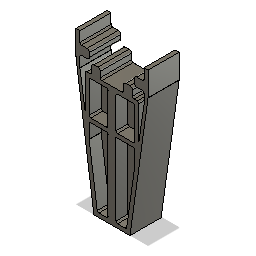
Tornado_Foot_75mm (Autodesk Fusion 360 design; units mm, degrees)
Autodesk Fusion 360 part; units mm, degrees
sketch "Sketch1" plane through (0, 0, 0) normal (0, 0, 1) x (1, 0, 0)
  line L0 (0, 0) -> (22.5, 0)
  line L1 (22.5, 0) -> (22.5, 95)
  line L2 (22.5, 95) -> (0, 95)
  line L3 (0, 95) -> (0, 0)
  line L4 (0, 95) -> (20, 95)
  line L5 (20, 95) -> (20, 75)
  line L6 (20, 75) -> (0, 75)
  line L7 (0, 75) -> (0, 95)
  line L8 (20, 95) -> (20, 85) construction
  line L9 (14, 87.75) -> (26, 87.75)
  line L10 (26, 87.75) -> (26, 82.25)
  line L11 (26, 82.25) -> (14, 82.25)
  line L12 (14, 82.25) -> (14, 87.75)
  line L13 (14, 87.75) -> (26, 82.25) construction
  line L14 (26, 87.75) -> (14, 82.25) construction
  line L15 (12.75, 81) -> (7.25, 81)
  line L16 (7.25, 81) -> (7.25, 69)
  line L17 (7.25, 69) -> (12.75, 69)
  line L18 (12.75, 69) -> (12.75, 81)
  line L19 (12.75, 81) -> (7.25, 69) construction
  line L20 (7.25, 81) -> (12.75, 69) construction
  line L21 (22.5, 80) -> (11.25, 0)
  line L22 (11.25, 0) -> (8.7744, 0.3481)
  line L23 (8.7744, 0.3481) -> (20, 75)
  line L24 (12.75, 75) -> (16.75, 75)
  line L25 (16.75, 75) -> (16.75, 53.3871)
  point P0 (20, 85)
  point P1 (10, 75)
  dimension "d1" = 5.5
  dimension "d2" = 12
  dimension "d3" = 12
  dimension "d4" = 5.5
  dimension "d5" = 22.5
  dimension "d6" = 95
  dimension "d7" = 20
  dimension "d8" = 20
  dimension "d28" = 2.5
  dimension "d29" = 4
  constraint horizontal L0
  constraint vertical L1
  constraint horizontal L2
  constraint vertical L3
  constraint coincident L0.start L3.end
  constraint horizontal L4
  constraint vertical L5
  constraint horizontal L6
  constraint vertical L7
  constraint midpoint L5 P0
  constraint perpendicular L9 L10
  constraint parallel L9 L11
  constraint parallel L10 L12
  constraint horizontal L9
  constraint coincident L13 P0
  constraint coincident L14 P0
  constraint coincident P0 L8.end
  constraint perpendicular L15 L16
  constraint parallel L15 L17
  constraint parallel L16 L18
  constraint horizontal L15
  constraint coincident L19 P1
  constraint coincident L20 P1
  constraint midpoint L6 P1
  constraint coincident L1 L21.start
  constraint midpoint L0 L21.end
  constraint perpendicular L21 L22
  constraint midpoint L18 L24.start
  constraint perpendicular L5 L24
  constraint vertical L25
  constraint coincident L23 L25.end
  measures "d1" distance of L9.end L10.end
  measures "d2" distance of L10.end L11.end
  measures "d3" distance of L15.end L16.end
  measures "d4" distance of L16.end L17.end
  measures "d5" distance of L0.start L0.end
  measures "d6" distance of L0.end L1.end
  measures "d7" distance of L4.end L5.end
  measures "d8" distance of L5.end L6.end
  measures "d28" distance of L21.end L22.end
  measures "d29" distance of L24.start L24.end
extrude "Extrude1" add sketch "Sketch1" along normal blind 10 contours L0 L3 L6 L16 L17 L18 L22 L23 L24 L25 | L1 L5 L11 L21 L22 L23 | L6 L15 L16 L18 | L6 L16 L17 L18 | L1 L5 L9 L11 | L1 L2 L5 L9 | L5 L9 L11 L12 makes body 1
fillet "Fillet1" [suppressed]
chamfer "Chamfer1" [suppressed]
mirror "Mirror1" about plane through (0, 75, 0) normal (1, 0, 0) of bodies 1 makes body 2
shell "Shell1" thickness 2.5 removed faces 1 at (5.5833, 42.7957, 10) on bodies 1
shell "Shell2" thickness 2.5 removed faces 1 at (-5.5833, 42.7957, 10) on bodies 2
combine "Combine1" operation add target body 2 tool bodies 1
sketch "Sketch2" plane through (0, 0, 10) normal (0, 0, 1) x (1, 0, 0)
  line L0 (-7.25, 81) -> (-12.75, 81)
  line L1 (-12.75, 81) -> (-12.75, 75)
  line L2 (-12.75, 75) -> (-16.75, 75)
  line L3 (-20, 75) -> (-20, 82.25)
  line L4 (-20, 82.25) -> (-14, 82.25)
  line L5 (-14, 82.25) -> (-14, 87.75)
  line L6 (-14, 87.75) -> (-20, 87.75)
  line L7 (-20, 87.75) -> (-20, 95)
  line L8 (-20, 95) -> (-22.5, 95)
  line L9 (-22.5, 95) -> (-22.5, 80)
  line L10 (-22.5, 80) -> (-11.25, 0)
  line L11 (-11.25, 0) -> (11.25, 0)
  line L12 (11.25, 0) -> (22.5, 80)
  line L13 (22.5, 80) -> (22.5, 95)
  line L14 (22.5, 95) -> (20, 95)
  line L15 (20, 95) -> (20, 87.75)
  line L16 (20, 87.75) -> (14, 87.75)
  line L17 (14, 87.75) -> (14, 82.25)
  line L18 (14, 82.25) -> (20, 82.25)
  line L19 (20, 82.25) -> (20, 75)
  line L20 (16.75, 75) -> (12.75, 75)
  line L21 (12.75, 75) -> (12.75, 81)
  line L22 (12.75, 81) -> (7.25, 81)
  line L23 (7.25, 81) -> (7.25, 75)
  line L24 (7.25, 75) -> (-7.25, 75)
  line L25 (-7.25, 75) -> (-7.25, 81)
  line L26 (0, 0) -> (0, 50) construction
  line L27 (17.391, 51.25) -> (-17.391, 51.25)
  line L28 (-17.391, 51.25) -> (-17.391, 48.75)
  line L29 (-17.391, 48.75) -> (17.391, 48.75)
  line L30 (17.391, 48.75) -> (17.391, 51.25)
  line L31 (17.391, 51.25) -> (-17.391, 48.75) construction
  line L32 (-17.391, 51.25) -> (17.391, 48.75) construction
  line L33 (-16.75, 75) -> (-16.75, 53.3871)
  line L34 (-16.75, 53.3871) -> (-20, 75)
  line L35 (20, 75) -> (16.75, 53.3871)
  line L36 (16.75, 53.3871) -> (16.75, 75)
  line L37 (-2.5, 72.5) -> (-2.5, 2.5)
  line L38 (-2.5, 2.5) -> (-9.077, 2.5)
  line L39 (-9.077, 2.5) -> (-14.25, 39.286)
  line L40 (-14.25, 39.286) -> (-14.25, 72.5)
  line L41 (-14.25, 72.5) -> (-10.25, 72.5)
  line L42 (-10.25, 72.5) -> (-10.25, 78.5)
  line L43 (-10.25, 78.5) -> (-9.75, 78.5)
  line L44 (-9.75, 78.5) -> (-9.75, 72.5)
  line L45 (-9.75, 72.5) -> (-2.5, 72.5)
  line L46 (2.5, 2.5) -> (2.5, 72.5)
  line L47 (2.5, 72.5) -> (9.75, 72.5)
  line L48 (9.75, 72.5) -> (9.75, 78.5)
  line L49 (9.75, 78.5) -> (10.25, 78.5)
  line L50 (10.25, 78.5) -> (10.25, 72.5)
  line L51 (10.25, 72.5) -> (14.25, 72.5)
  line L52 (14.25, 72.5) -> (14.25, 39.286)
  line L53 (14.25, 39.286) -> (9.077, 2.5)
  line L54 (9.077, 2.5) -> (2.5, 2.5)
  line L55 (20, 85.25) -> (20, 84.75)
  line L56 (20, 84.75) -> (16.5, 84.75)
  line L57 (16.5, 84.75) -> (16.5, 85.25)
  line L58 (16.5, 85.25) -> (20, 85.25)
  line L59 (-20, 84.75) -> (-20, 85.25)
  line L60 (-20, 85.25) -> (-16.5, 85.25)
  line L61 (-16.5, 85.25) -> (-16.5, 84.75)
  line L62 (-16.5, 84.75) -> (-20, 84.75)
  point P0 (0, 50)
  dimension "d16" = 50
  dimension "d17" = 2.5
  constraint vertical L26
  constraint coincident L26.start origin
  constraint perpendicular L27 L28
  constraint parallel L27 L29
  constraint parallel L28 L30
  constraint horizontal L27
  constraint coincident L31 P0
  constraint coincident L32 P0
  constraint coincident P0 L26.end
  measures "d16" distance of L26.start P0
  measures "d17" distance of L27.end L28.end
extrude "Extrude2" add sketch "Sketch2" against normal up to surface (10 mm away) contours L0 L1 L2 L3 L4 L5 L6 L7 L8 L9 L10 L11 L12 L13 L14 L15 L16 L17 L18 L19 L20 L21 L22 L23 L24 L25 L33 L34 L35 L36 | L27 L29 L46 L52 | L27 L29 L37 L40 | L55 L56 L57 L58 | L59 L60 L61 L62 bodies 2
fillet "Fillet4" radius 1 17 edges at (-14.25, 72.5, 6.25) (2.5, 72.5, 6.25) (-2.5, 72.5, 6.25) (14.25, 72.5, 6.25) (-14.25, 51.25, 6.25) (-2.5, 51.25, 6.25) (2.5, 51.25, 6.25) (14.25, 51.25, 6.25) (-14.25, 39.286, 6.25) (-14.25, 48.75, 6.25) (-2.5, 48.75, 6.25) (14.25, 48.75, 6.25) (14.25, 39.286, 6.25) (-9.077, 2.5, 6.25) (-2.5, 2.5, 6.25) (2.5, 2.5, 6.25) (9.077, 2.5, 6.25) on bodies 2
extrude "Extrude4" add 2 faces at (-10.0833, 78.5, 5) (9.9167, 78.5, 7.5) along direction (0, -1, 0) blind 6 on bodies 2 bodies 2
mirror "Mirror2" about plane through (0, 0, 0) normal (0, 0, -1) of bodies 2 makes body 3
combine "Combine2" operation add target body 2 tool bodies 3
fillet "Fillet2" radius 1.5 8 edges at (14, 87.75, 0) (12.75, 81, 0) (14, 82.25, 0) (7.25, 81, 0) (-7.25, 81, 0) (-12.75, 81, 0) (-14, 82.25, 0) (-14, 87.75, 0) on bodies 2
fillet "Fillet3" radius 1 14 edges at (16.75, 75, 0) (22.5, 80, 0) (-20, 75, 0) (-22.5, 80, 0) (20, 75, 0) (-16.75, 75, 0) (12.75, 75, 0) (7.25, 75, 0) (-7.25, 75, 0) (-12.75, 75, 0) (-20, 87.75, 0) (-20, 82.25, 0) (20, 87.75, 0) (20, 82.25, 0) on bodies 2
chamfer "Chamfer2" distance 0.6 angle 45 52 edges at (16.8701, 39.9654, -10) (22.4976, 80.0002, -10) (22.5, 87.535, -10) (20, 91.875, -10) (19.7071, 88.0429, -10) (17.25, 87.75, -10) (14.4393, 87.3107, -10) (14, 85, -10) (14.4393, 82.6893, -10) (17.25, 82.25, -10) (19.7071, 81.9571, -10) (20, 78.1624, -10) (19.9972, 75.0002, -10) (18.3694, 64.1566, -10) (16.75, 63.6936, -10) (16.4571, 74.7071, -10) (14.75, 75, -10) (13.0429, 75.2929, -10) (12.75, 77.75, -10) (12.3107, 80.5607, -10) (10, 81, -10) (7.6893, 80.5607, -10) (7.25, 77.75, -10) (6.9571, 75.2929, -10) (0, 75, -10) (-6.9571, 75.2929, -10) (-7.25, 77.75, -10) (-7.6893, 80.5607, -10) (-10, 81, -10) (-12.3107, 80.5607, -10) (-12.75, 77.75, -10) (-13.0429, 75.2929, -10) (-14.75, 75, -10) (-16.4571, 74.7071, -10) (-16.75, 63.6936, -10) (-16.8701, 39.9654, -10) (-22.4976, 80.0002, -10) (-22.5, 87.535, -10) (0, 0, -10) (-20, 91.875, -10) (-19.7071, 88.0429, -10) (-17.25, 87.75, -10) (-14.4393, 87.3107, -10) (-14, 85, -10) (-14.4393, 82.6893, -10) (-17.25, 82.25, -10) (-19.7071, 81.9571, -10) (-20, 78.1624, -10) (-19.9972, 75.0002, -10) (-18.3694, 64.1566, -10) (21.25, 95, -10) (-21.25, 95, -10) on bodies 2
